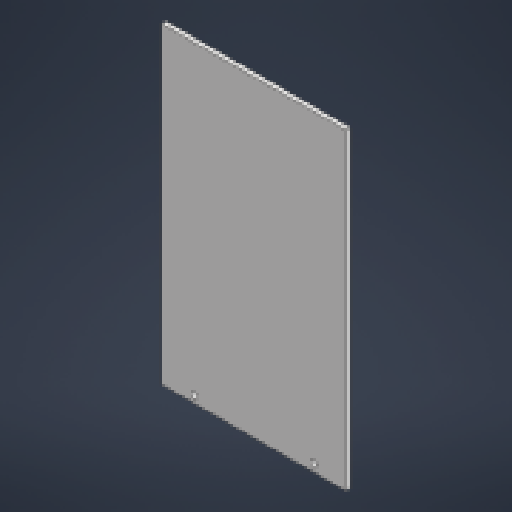
# Autodesk Inventor part: Shelf1
Saved by Autodesk Inventor 2023.4 (Build 274418000, 418)
## iProperties
Created: 2025-10-22
Part Number: Shelf1
Material: Generic
Document SubType Name: Modeling
Designer: Malthe Sennels
Density: 1 g/cm^3
Appearance: Polycarbonate - Clear
Author: Malthe Sennels
Autodesk Inventor part; units mm, degrees
ref_plane "YZ Plane" through (0, 0, 0) normal (1, 0, 0) x (0, 1, 0)
ref_plane "XZ Plane" through (0, 0, 0) normal (0, 1, 0) x (-1, 0, 0)
ref_plane "XY Plane" through (0, 0, 0) normal (0, 0, 1) x (1, 0, 0)
sketch "Sketch1" plane through (0, 0, 0) normal (0, 0, 1) x (1, 0, 0)
  line L0 (-120, 25) -> (-122, 25) construction
  line L1 (-122, 0) -> (-122, 25) projected
  line L2 (-110, 0) -> (-122, 0) projected
  line L3 (-120, 10) -> (-110, 0) construction
  line L4 (-120, 10) -> (-120, 18.3797) construction
  line L5 (-80.5845, 0) -> (-120, 18.3797) construction
  line L6 (-66.3873, 0) -> (-80.5845, 0) projected
  line L7 (-120, 25) -> (-66.3873, 0) construction
  line L8 (2, 25) -> (0, 25) construction
  line L9 (-53.6127, 0) -> (0, 25) construction
  line L10 (-39.4155, 0) -> (-53.6127, 0) projected
  line L11 (0, 18.3797) -> (-39.4155, 0) construction
  line L12 (0, 10) -> (0, 18.3797) construction
  line L13 (-10, 0) -> (0, 10) construction
  line L14 (2, 0) -> (-10, 0) projected
  line L15 (2, 0) -> (2, 25) projected
  line L16 (2, 0) -> (-122, 0)
  line L17 (-122, 0) -> (-122, 210)
  line L18 (-122, 210) -> (2, 210)
  line L19 (2, 210) -> (2, 0)
  circle A0 centre (-100, 5) radius 2.25 projected
  circle A1 centre (-20, 5) radius 2.25 projected
  point P0 (0, 0)
  point P1 (2, 25)
  dimension "d0" = 124
  dimension "d1" = 210
  constraints: 8 end point, 2 parallel, 1 horizontal, 1 perpendicular
  measures "d0" distance of L17.end L18.end
  measures "d1" distance from line of L2.start L18
extrude "Extrusion1" add sketch "Sketch1" along normal blind 3
body "Solid1"
